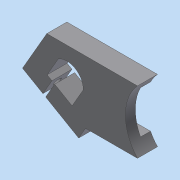
# Autodesk Inventor part: motormount3
Saved by Autodesk Inventor 2017 (Build 210142000, 142)
## iProperties
Created: 2015-12-12
Part Number: motormount3
Material: Generic
Document SubType Name: Modeling
Designer: JoshuaYuan
Density: 1 g/cm^3
Appearance: Default
Author: JoshuaYuan
Autodesk Inventor part; units mm, degrees
ref_plane "YZ Plane" through (0, 0, 0) normal (1, 0, 0) x (0, 1, 0)
ref_plane "XZ Plane" through (0, 0, 0) normal (0, 1, 0) x (-1, 0, 0)
ref_plane "XY Plane" through (0, 0, 0) normal (0, 0, 1) x (1, 0, 0)
sketch "Sketch1" plane through (0, 0, 0) normal (0, 0, 1) x (1, 0, 0)
  circle A0 centre (67.04, 0) radius 29.5
  line L0 (-4.9819, 9.659) -> (-12.0939, -2.6593)
  line L1 (3.7439, -11.8033) -> (10.8559, 0.515)
  arc A1 (10.8559, 0.515) -> (-4.9819, 9.659) centre (0.4451, 0.7709) ccw
  line L2 (-52.5571, 0) -> (121.3895, 0) projected
  line L3 (-12.2744, 19.8882) -> (-27.7076, -6.843)
  line L4 (-27.7076, -6.843) -> (-14.7443, -14.3274)
  line L5 (-12.2744, 19.8882) -> (45.2522, 19.8882)
  line L6 (0, -41.3) -> (0, 41.3) projected
  line L7 (40.8299, 13.5382) -> (17.0809, 13.5382)
  line L8 (13.9059, 10.3632) -> (13.9059, -10.3632)
  line L9 (17.0809, -13.5382) -> (40.8299, -13.5382)
  arc A2 (17.0809, 13.5382) -> (13.9059, 10.3632) centre (17.0809, 10.3632) ccw
  arc A3 (13.9059, -10.3632) -> (17.0809, -13.5382) centre (17.0809, -10.3632) ccw
  line L10 (-9.0293, -4.4287) -> (-14.7443, -14.3274)
  line L11 (-13.0122, -15.3274) -> (-7.2972, -5.4287)
  line L12 (-13.0122, -15.3274) -> (7.9276, -27.417)
  line L13 (-12.0939, -2.6593) -> (-9.0293, -4.4287)
  line L14 (-7.2972, -5.4287) -> (3.7439, -11.8033)
  line L15 (7.9276, -27.417) -> (12.2744, -19.8882)
  line L16 (12.2744, -19.8882) -> (45.2522, -19.8882)
  circle A4 centre (0, 0) radius 3.975
  circle A5 centre (19.4307, 7.7635) radius 2.0193
  point P0 (0, 0)
  point P1 (13.9059, 13.5382)
  point P2 (13.9059, -13.5382)
  dimension "d22" = 12.7
  dimension "d25" = 19.05
  dimension "d2" = 59
  dimension "d3" = 14.224
  dimension "d4" = 18.288
  dimension "d11" = 11.43
  dimension "d45" = 3.175
  dimension "d48" = 2
  dimension "d56" = 10.414
  dimension "d57" = 26.924
  dimension "d58" = 11.43
  dimension "d59" = 30
  dimension "d69" = 20.7264
  dimension "d88" = 6.35
  dimension "d89" = 6.35
  dimension "d90" = 11.43
  dimension "d91" = 7.95
  dimension "d92" = 8.35
  dimension "d93" = 9.144
  dimension "d94" = 4.0386
  constraints: 30 end point, 10 point on circle, 7 perpendicular, 6 centre point, 5 point on line, 4 parallel, 4 tangent, 3 horizontal, 2 collinear, 1 coincident, 1 equal radius, 1 vertical, 1 other
  measures "d2" diameter of A0
  measures "d3" distance of L1.start L1.end
  measures "d4" distance of L0.end L1.start
  measures "d11" distance between parallel lines of L3 L0
  measures "d45" radius of A2
  measures "d48" distance between parallel lines of L10 L11
  measures "d56" radius of A1
  measures "d57" distance from line of L8 L9.end
  measures "d58" distance between parallel lines of L4 L13
  measures "d59" angle of L2 L13
  measures "d69" distance of L8.start L8.end
  measures "d88" distance between parallel lines of L7 L5
  measures "d89" distance between parallel lines of L16 L9
  measures "d90" distance between parallel lines of L15 L1
  measures "d91" diameter of A4
  measures "d92" distance from line of L14 A4.centre
  measures "d93" distance from line of L0 A4.centre
  measures "d94" diameter of A5
extrude "plate" add sketch "Sketch1" along normal blind 12.7 contours A0 L7 A2 L8 L2 L1 A1 L6 L5 | L16 L15 L12 L6 L14 L1 L2 L8 A3 L9 A0 | L2 L8 A2 L7 A0 | A0 L9 A3 L8 L2 | L6 A1 L0 L2 L3 L5 | L2 L0 L13 L10 L4 L3 | L12 L11 L14 L6 | A5
extrude "cut out" cut sketch "Sketch1" along normal blind 6.35 contours L2 L8 A2 L7 A0 | A0 L9 A3 L8 L2 | A5
extrude "tension holes" [suppressed]
ref_plane "Work Plane1" through (14.1221, 4.6482, 12.7) normal (-0.8660254, 0.5, 0) x (0, 0, 1)
sketch "Sketch2" plane through (-12.2744, 19.8882, 12.7) normal (-0.8660254, 0.5, 0) x (0, 0, 1)
  line L0 (-12.7, -19.4365) -> (0, -19.4365) projected
  line L1 (-12.7, -30.8665) -> (0, -30.8665) projected
  line L2 (-6.35, -19.4365) -> (-6.35, -30.8665) construction
  circle A0 centre (-6.35, -25.1515) radius 2.3813
  dimension "d60" = 4.7625
  constraints: 3 midpoint, 2 end point, 1 centre point
  measures "d60" diameter of A0
extrude "clamp screw" cut sketch "Sketch2" against normal through all
body "Solid1"
